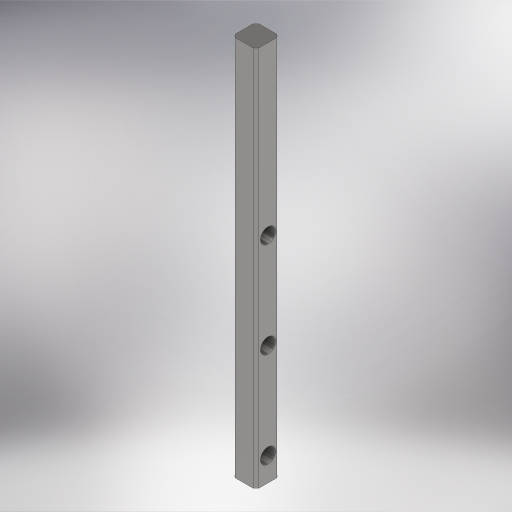
# Autodesk Inventor part: assist
Saved by Autodesk Inventor 2023 (Build 270158000, 158)
## iProperties
Created: 2023-01-16
Part Number: assist
Material: Stainless Steel
Document SubType Name: Modeling
Designer: aaron
Density: 8 g/cm^3
Appearance: Semi-Polished
Author: aaron
Autodesk Inventor part; units mm, degrees
ref_plane "YZ Plane" through (0, 0, 0) normal (1, 0, 0) x (0, 1, 0)
ref_plane "XZ Plane" through (0, 0, 0) normal (0, 1, 0) x (-1, 0, 0)
ref_plane "XY Plane" through (0, 0, 0) normal (0, 0, 1) x (1, 0, 0)
sketch "Sketch1" plane through (0, 0, 0) normal (0, 1, 0) x (-1, 0, 0)
  line L0 (-3.175, -3.175) -> (3.175, -3.175)
  line L1 (3.175, -3.175) -> (3.175, 3.175)
  line L2 (3.175, 3.175) -> (-3.175, 3.175)
  line L3 (-3.175, 3.175) -> (-3.175, -3.175)
  line L4 (-3.175, -3.175) -> (3.175, 3.175) construction
  line L5 (3.175, -3.175) -> (-3.175, 3.175) construction
  circle A0 centre (0, 0) radius 3.9688
  point P0 (2.3812, -3.175)
  point P1 (3.175, -2.3812)
  point P2 (3.175, 2.3812)
  point P3 (2.3812, 3.175)
  point P4 (-2.3812, 3.175)
  point P5 (-3.175, 2.3812)
  point P6 (-3.175, -2.3812)
  point P7 (-2.3812, -3.175)
  dimension "d0" = 6.35
  dimension "d1" = 6.35
  dimension "d2" = 7.9375
  constraints: 12 end point, 2 midpoint, 2 parallel, 1 centre point, 1 coincident, 1 horizontal, 1 perpendicular
  measures "d0" distance of L2.end L1.end
  measures "d1" distance of L1.end L0.end
  measures "d2" diameter of A0
extrude "Extrusion1" add sketch "Sketch1" along normal blind 101.6 contours A0 L3 L2 L1 L0
sketch "Sketch2" plane through (3.175, 0, 2.3812) normal (1, 0, 0) x (0, 0, -1)
  circle A0 centre (2.3812, 6.35) radius 1.9844
  line L0 (0, 0) -> (4.7625, 0) projected
  line L1 (-0.7938, 0) -> (-0.7938, 101.6) projected
  circle A1 centre (2.3812, 19.05) radius 1.9844
  circle A2 centre (2.3812, 31.75) radius 1.9844
  circle A3 centre (2.3812, 44.45) radius 1.9844
  circle A4 centre (2.3812, 57.15) radius 1.9844
  point P0 (2.3812, 0)
  dimension "d5" = 3.9688
  dimension "d6" = 6.35
  dimension "d9" = 12.7
  constraints: 5 centre point, 1 vertical, 8 other
  measures "d5" diameter of A0
  measures "d6" distance from line of L0 A0.centre
  measures "d9" distance of A0.centre A1.centre
extrude "Extrusion2" cut sketch "Sketch2" against normal blind 101.6 contours A0 | A2 | A4
body "Solid1"
